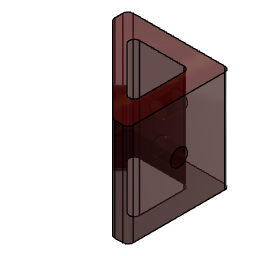
A shake table - 2020 extrusion cross connector (Autodesk Fusion 360 design; units mm, degrees)
Autodesk Fusion 360 part; units mm, degrees
sketch "Sketch1" plane through (0, 0, 0) normal (0, 1, 0) x (1, 0, 0)
  line L0 (0, 0) -> (-100, 0) construction
  line L1 (-100, 0) -> (-100, -100) construction
  line L2 (-100, -100) -> (0, -100) construction
  line L3 (0, -100) -> (0, 0) construction
  line L4 (10, 20) -> (-110, 20)
  line L5 (-120, 10) -> (-120, -110)
  line L6 (-110, -120) -> (10, -120)
  line L7 (20, -110) -> (20, 10)
  circle A0 centre (0, 0) radius 1.65
  circle A1 centre (-100, 0) radius 1.65
  circle A2 centre (0, -100) radius 1.65
  circle A3 centre (-100, -100) radius 1.65
  arc A4 (10, -120) -> (20, -110) centre (10, -110) ccw
  arc A5 (-120, -110) -> (-110, -120) centre (-110, -110) ccw
  arc A6 (-110, 20) -> (-120, 10) centre (-110, 10) ccw
  arc A7 (20, 10) -> (10, 20) centre (10, 10) ccw
  dimension "d1" = 100
  dimension "d2" = 100
  dimension "d4" = 3.3
  dimension "d7" = -100
  dimension "d8" = -100
  dimension "d9" = 10
  constraint horizontal L0
  constraint vertical L1
  constraint horizontal L2
  constraint vertical L3
  constraint coincident L0.start L3.end
  constraint parallel L0 L4
  constraint parallel L1 L5
  constraint parallel L2 L6
  constraint parallel L3 L7
  constraint tangent L6 A4
  constraint tangent L7 A4
  constraint tangent L5 A5
  constraint tangent L6 A5
  constraint equal A4 A5
  constraint tangent L4 A6
  constraint tangent L5 A6
  constraint equal A4 A6
  constraint tangent L4 A7
  constraint tangent L7 A7
  constraint equal A4 A7
  measures "d1" distance of L0.start L0.end
  measures "d2" distance of L0.start L2.end
  measures "d4" diameter of A0
  measures "d9" radius of A4
extrude "Extrude1" add sketch "Sketch1" along normal blind 7 makes body 1
sketch "Sketch2" plane through (0, 7, 0) normal (0, 1, 0) x (-1, 0, 0)
  circle A0 centre (0, 0) radius 1.65
  circle A1 centre (100, 100) radius 1.65
  circle A2 centre (0, 100) radius 1.65
  circle A3 centre (100, 0) radius 1.65
  arc A4 (-20, -10) -> (-10, -20) centre (-10, -10) ccw
  line L0 (-10, -20) -> (110, -20)
  arc A5 (110, -20) -> (120, -10) centre (110, -10) ccw
  line L1 (120, -10) -> (120, 110)
  arc A6 (120, 110) -> (110, 120) centre (110, 110) ccw
  line L2 (110, 120) -> (-10, 120)
  arc A7 (-10, 120) -> (-20, 110) centre (-10, 110) ccw
  line L3 (-20, 110) -> (-20, -10)
  circle A8 centre (0, 0) radius 2.8
  circle A9 centre (100, 0) radius 2.8
  circle A10 centre (0, 100) radius 2.8
  circle A11 centre (100, 100) radius 2.8
  dimension "d12" = 5.6
  dimension "d15" = 100
  dimension "d16" = 100
  constraint coincident A0.centre A8.centre
  measures "d12" diameter of A8
extrude "Extrude2" cut sketch "Sketch2" against normal blind 3 contours A8 | A9 | A10 | A11 bodies 1
sketch "Sketch3" plane through (0, 0, 0) normal (0, 1, 0) x (1, 0, 0)
  line L0 (-1, 0) -> (-19, 0)
  line L1 (0, -19) -> (0, -1)
  line L2 (-1, -20) -> (-2.5858, -20)
  line L3 (-20, -1) -> (-20, -2.5858)
  line L4 (-19.7071, -3.2929) -> (-3.2929, -19.7071)
  line L5 (-14.4645, -5.7071) -> (-5.7071, -14.4645)
  line L6 (-5, -4) -> (-13.7574, -4)
  line L7 (-4, -13.7574) -> (-4, -5)
  arc A0 (-1, -20) -> (0, -19) centre (-1, -19) ccw
  arc A1 (-3.2929, -19.7071) -> (-2.5858, -20) centre (-2.5858, -19) ccw
  arc A2 (0, -1) -> (-1, 0) centre (-1, -1) ccw
  arc A3 (-19, 0) -> (-20, -1) centre (-19, -1) ccw
  arc A4 (-20, -2.5858) -> (-19.7071, -3.2929) centre (-19, -2.5858) ccw
  arc A5 (-5.7071, -14.4645) -> (-4, -13.7574) centre (-5, -13.7574) ccw
  arc A6 (-4, -5) -> (-5, -4) centre (-5, -5) ccw
  arc A7 (-13.7574, -4) -> (-14.4645, -5.7071) centre (-13.7574, -5) ccw
  point P0 (-20, 0)
  point P1 (0, -20)
  point P2 (-3, -20)
  point P3 (-20, -3)
  dimension "d19" = 20
  dimension "d20" = 20
  dimension "d23" = 3
  dimension "d24" = 3
  dimension "d26" = 1
  dimension "d27" = 1
  dimension "d30" = 2
  constraint horizontal L0
  constraint vertical L1
  constraint perpendicular L1 L2
  constraint perpendicular L0 L3
  constraint coincident P1 L2
  constraint coincident P1 L1
  constraint tangent L2 A0
  constraint tangent L1 A0
  constraint coincident P2 L2
  constraint coincident P2 L4
  constraint tangent L2 A1
  constraint tangent L4 A1
  constraint equal A0 A1
  constraint coincident origin L1
  constraint coincident origin L0
  constraint tangent L1 A2
  constraint tangent L0 A2
  constraint equal A0 A2
  constraint coincident P0 L3
  constraint coincident P0 L0
  constraint tangent L3 A3
  constraint tangent L0 A3
  constraint equal A0 A3
  constraint coincident P3 L4
  constraint coincident P3 L3
  constraint tangent L4 A4
  constraint tangent L3 A4
  constraint equal A0 A4
  constraint parallel L4 L5
  constraint parallel L0 L6
  constraint parallel L1 L7
  constraint tangent L5 A5
  constraint tangent L7 A5
  constraint tangent L6 A6
  constraint tangent L7 A6
  constraint equal A5 A6
  constraint tangent L5 A7
  constraint tangent L6 A7
  constraint equal A5 A7
  measures "d19" distance of origin P0
  measures "d20" distance of origin P1
  measures "d23" distance of P1 P2
  measures "d24" distance of P0 P3
  measures "d26" radius of A0
  measures "d27" radius of A5
  measures "d30" distance of L4 L5
extrude "Extrude3" add sketch "Sketch3" along normal blind 20 separate body makes body 2
sketch "Sketch4" plane through (0, 0, 0) normal (0, 0, -1) x (-1, 0, 0)
  line L0 (1, 0) -> (19, 0)
  line L1 (19, 0) -> (19, 20)
  line L2 (19, 20) -> (1, 20)
  line L3 (1, 20) -> (1, 0)
  circle A0 centre (10, 10) radius 1.65
  dimension "d31" = 3.3
  measures "d31" diameter of A0
extrude "Extrude5" cut sketch "Sketch4" against normal blind 30 contours A0 bodies 2
sketch "Sketch5" plane through (0, 0, 0) normal (1, 0, 0) x (0, 0, -1)
  line L0 (-19, 0) -> (-1, 0)
  line L1 (-1, 0) -> (-1, 20)
  line L2 (-1, 20) -> (-19, 20)
  line L3 (-19, 20) -> (-19, 0)
  circle A0 centre (-10, 10) radius 1.65
  dimension "d34" = 3.3
  measures "d34" diameter of A0
extrude "Extrude6" cut sketch "Sketch5" against normal blind 49 contours A0 bodies 2
sketch "Sketch6" plane through (-11.5, 0, 11.5) normal (-0.707107, 0, 0.707107) x (0.707107, 0, 0.707107)
  line L0 (-11.6066, 0) -> (11.6066, 0)
  line L1 (11.6066, 0) -> (11.6066, 20)
  line L2 (11.6066, 20) -> (-11.6066, 20)
  line L3 (-11.6066, 20) -> (-11.6066, 0)
  ellipse E0 centre (-2.1213, 10) end of major axis (-4.4548, 10) minor radius 1.65 (0, 10.6874) -> (0, 9.3126) ccw
  ellipse E1 centre (2.1213, 10) end of major axis (-0.2121, 10) minor radius 1.65 (0, 9.3126) -> (0, 10.6874) ccw
  circle A0 centre (0, 10) radius 6
  dimension "d37" = 12
  measures "d37" diameter of A0
extrude "Extrude7" cut sketch "Sketch6" against normal blind 3 contours E0 E1 | A0 bodies 2
extrude "Extrude4" [suppressed]
hidden bodies 1
